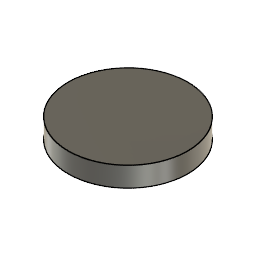
Lead Screw Head (Autodesk Fusion 360 design; units mm, degrees)
part number: 2026-04-26-20-37-26-178
Autodesk Fusion 360 part; units mm, degrees
sketch "Sketch6" plane through (0, 0, 0) normal (0, 0, 1) x (1, 0, 0)
  circle A0 centre (0, 0) radius 30
  dimension "d20" = 60
  constraint coincident A0.centre origin
  measures "d20" diameter of A0
extrude "Extrude5" add sketch "Sketch6" along normal blind 10
